Autodesk Inventor part; units mm, degrees
note: some values were not read from the file. Chosen so that the rebuilt part matches the saved one: bend side of "曲げパーツ2".
(part 2 of 2)
sketch "スケッチ2" plane through (0, 0, 0) normal (0, 0, -1) x (-1, 0, 0)
  line L0 (-121.1595, -137.1852) -> (-101.7935, -131.1964) projected
  arc A0 (-101.7935, -131.1964) -> (-101.8327, -129.2745) centre (-102.089, -130.2411) ccw projected
  line L1 (-101.8327, -129.2745) -> (-140.7437, -118.9579) projected
  arc A1 (-140.7437, -118.9579) -> (-142, -119.9245) centre (-141, -119.9245) ccw projected
  line L2 (-142, -119.9245) -> (-142, -142.2739) projected
  arc A2 (-142, -142.2739) -> (-140.7046, -143.2293) centre (-141, -142.2739) ccw projected
  line L3 (-140.7046, -143.2293) -> (-133.575, -141.0246) projected
  arc A3 (-133.575, -141.0246) -> (-132.8964, -140.2954) centre (-133.8705, -140.0692) ccw projected
  arc A4 (-126.6, -138) -> (-132.8964, -140.2954) centre (-129, -141.2) ccw projected
  arc A5 (-126.6, -138) -> (-126, -138.2) centre (-126, -137.2) ccw projected
  line L4 (-126, -138.2) -> (-125, -138.2) projected
  arc A6 (-125, -138.2) -> (-124.4, -138) centre (-125, -137.2) ccw projected
  arc A7 (-121.5639, -137.2238) -> (-124.4, -138) centre (-122, -141.2) ccw projected
  arc A8 (-121.5639, -137.2238) -> (-121.1595, -137.1852) centre (-121.4549, -136.2298) ccw projected
  line L5 (-125, 4) -> (-126, 4) projected
  arc A9 (-126, 4) -> (-126.6, 3.8) centre (-126, 3) ccw projected
  arc A10 (-132.8927, 6.0797) -> (-126.6, 3.8) centre (-129, 7) ccw projected
  arc A11 (-132.8927, 6.0797) -> (-133.5686, 6.8044) centre (-133.8659, 5.8496) ccw projected
  line L6 (-133.5686, 6.8044) -> (-140.7028, 9.0252) projected
  arc A12 (-140.7028, 9.0252) -> (-142, 8.0704) centre (-141, 8.0704) ccw projected
  line L7 (-142, 8.0704) -> (-142, -14.2755) projected
  arc A13 (-142, -14.2755) -> (-140.7437, -15.2421) centre (-141, -14.2755) ccw projected
  line L8 (-140.7437, -15.2421) -> (-101.9774, -4.9639) projected
  arc A14 (-101.9774, -4.9639) -> (-101.9364, -3.0425) centre (-102.2336, -3.9973) ccw projected
  line L9 (-101.9364, -3.0425) -> (-121.2641, 2.9741) projected
  arc A15 (-121.2641, 2.9741) -> (-121.6491, 3.0154) centre (-121.5614, 2.0193) ccw projected
  arc A16 (-124.4, 3.8) -> (-121.6491, 3.0154) centre (-122, 7) ccw projected
  arc A17 (-124.4, 3.8) -> (-125, 4) centre (-125, 3) ccw projected
  line L10 (-128.2505, -119.1666) -> (-93.3393, -128.4227) projected
  arc A18 (-93.3393, -128.4227) -> (-92.7876, -128.4114) centre (-93.0831, -127.4561) ccw projected
  line L11 (-92.7876, -128.4114) -> (-62.8561, -119.1554) projected
  arc A19 (-62.8561, -119.1554) -> (-63.1515, -117.2) centre (-63.1515, -118.2) ccw projected
  line L12 (-63.1515, -117.2) -> (-127.9942, -117.2) projected
  arc A20 (-127.9942, -117.2) -> (-128.2505, -119.1666) centre (-127.9942, -118.2) ccw projected
  line L13 (-127.9942, -17) -> (-63.676, -17) projected
  arc A21 (-63.676, -17) -> (-63.3788, -15.0452) centre (-63.676, -16) ccw projected
  line L14 (-63.3788, -15.0452) -> (-92.9626, -5.836) projected
  arc A22 (-92.9626, -5.836) -> (-93.5161, -5.8242) centre (-93.2598, -6.7908) ccw projected
  line L15 (-93.5161, -5.8242) -> (-128.2505, -15.0334) projected
  arc A23 (-128.2505, -15.0334) -> (-127.9942, -17) centre (-127.9942, -16) ccw projected
  line L16 (-52.2563, 5.1151) -> (-84.4313, -3.4155) projected
  arc A24 (-84.4313, -3.4155) -> (-84.4723, -5.337) centre (-84.1751, -4.3821) ccw projected
  line L17 (-84.4723, -5.337) -> (-52.2972, -15.3528) projected
  arc A25 (-52.2972, -15.3528) -> (-51, -14.398) centre (-52, -14.398) ccw projected
  line L18 (-51, -14.398) -> (-51, 4.1485) projected
  arc A26 (-51, 4.1485) -> (-52.2563, 5.1151) centre (-52, 4.1485) ccw projected
  line L19 (-51, -138.3485) -> (-51, -119.9851) projected
  arc A27 (-51, -119.9851) -> (-52.2954, -119.0297) centre (-52, -119.9851) ccw projected
  line L20 (-52.2954, -119.0297) -> (-84.2666, -128.9165) projected
  arc A28 (-84.2666, -128.9165) -> (-84.2275, -130.8385) centre (-83.9712, -129.8719) ccw projected
  line L21 (-84.2275, -130.8385) -> (-52.2563, -139.3151) projected
  arc A29 (-52.2563, -139.3151) -> (-51, -138.3485) centre (-52, -138.3485) ccw projected
  arc A30 (-86.4, 3.8) -> (-80.0808, 6.2) centre (-84, 7) ccw projected
  arc A31 (-86.4, 3.8) -> (-87, 4) centre (-87, 3) ccw projected
  line L22 (-87, 4) -> (-88, 4) projected
  arc A32 (-88, 4) -> (-88.6, 3.8) centre (-88, 3) ccw projected
  arc A33 (-95, 7) -> (-88.6, 3.8) centre (-91, 7) ccw projected
  line L23 (-95, 7) -> (-95, 10) projected
  arc A34 (-95, 10) -> (-96, 11) centre (-96, 10) ccw projected
  line L24 (-96, 11) -> (-117, 11) projected
  arc A35 (-117, 11) -> (-118, 10) centre (-117, 10) ccw projected
  line L25 (-118, 10) -> (-118, 7) projected
  arc A36 (-118.1024, 6.1007) -> (-118, 7) centre (-122, 7) ccw projected
  arc A37 (-118.1024, 6.1007) -> (-117.4252, 4.9211) centre (-117.128, 5.8759) ccw projected
  line L26 (-117.4252, 4.9211) -> (-93.4461, -2.5435) projected
  arc A38 (-93.4461, -2.5435) -> (-92.8926, -2.5553) centre (-93.1489, -1.5887) ccw projected
  line L27 (-92.8926, -2.5553) -> (-64.2705, 5.0334) projected
  arc A39 (-64.2705, 5.0334) -> (-64.5268, 7) centre (-64.5268, 6) ccw projected
  line L28 (-64.5268, 7) -> (-79.101, 7) projected
  arc A40 (-79.101, 7) -> (-80.0808, 6.2) centre (-79.101, 6) ccw projected
  line L29 (-117, -145.2) -> (-96, -145.2) projected
  arc A41 (-96, -145.2) -> (-95, -144.2) centre (-96, -144.2) ccw projected
  line L30 (-95, -144.2) -> (-95, -141.2) projected
  arc A42 (-88.6, -138) -> (-95, -141.2) centre (-91, -141.2) ccw projected
  arc A43 (-88.6, -138) -> (-88, -138.2) centre (-88, -137.2) ccw projected
  line L31 (-88, -138.2) -> (-87, -138.2) projected
  arc A44 (-87, -138.2) -> (-86.4, -138) centre (-87, -137.2) ccw projected
  arc A45 (-80.0808, -140.4) -> (-86.4, -138) centre (-84, -141.2) ccw projected
  arc A46 (-80.0808, -140.4) -> (-79.101, -141.2) centre (-79.101, -140.2) ccw projected
  line L32 (-79.101, -141.2) -> (-64.5268, -141.2) projected
  arc A47 (-64.5268, -141.2) -> (-64.2705, -139.2334) centre (-64.5268, -140.2) ccw projected
  line L33 (-64.2705, -139.2334) -> (-92.7208, -131.6903) projected
  arc A48 (-92.7208, -131.6903) -> (-93.2725, -131.7015) centre (-92.9771, -132.6569) ccw projected
  line L34 (-93.2725, -131.7015) -> (-117.413, -139.1668) projected
  arc A49 (-117.413, -139.1668) -> (-118.094, -140.3377) centre (-117.1176, -140.1221) ccw projected
  arc A50 (-118, -141.2) -> (-118.094, -140.3377) centre (-122, -141.2) ccw projected
  line L35 (-118, -141.2) -> (-118, -144.2) projected
  arc A51 (-118, -144.2) -> (-117, -145.2) centre (-117, -144.2) ccw projected
  line L36 (-123, -169.2) -> (-122, -169.2) projected
  arc A52 (-122, -169.2) -> (-121, -168.2) centre (-122, -168.2) ccw projected
  line L37 (-121, -168.2) -> (-121, -166.2) projected
  arc A53 (-121, -166.2) -> (-120.7896, -164.437) centre (-121.3519, -165.264) ccw projected
  line L38 (-120.7896, -164.437) -> (-128.9377, -158.8963) projected
  arc A54 (-128.9377, -158.8963) -> (-130.0623, -158.8963) centre (-129.5, -159.7232) ccw projected
  line L39 (-130.0623, -158.8963) -> (-135.1564, -162.3603) projected
  arc A55 (-135.1564, -162.3603) -> (-135.577, -163.3713) centre (-134.5941, -163.1872) ccw projected
  arc A56 (-135.575, -165.0182) -> (-135.577, -163.3713) centre (-140, -164.2) ccw projected
  arc A57 (-135.575, -165.0182) -> (-134.5917, -166.2) centre (-134.5917, -165.2) ccw projected
  line L40 (-134.5917, -166.2) -> (-134, -166.2) projected
  arc A58 (-134, -166.2) -> (-133.4, -166) centre (-134, -165.2) ccw projected
  arc A59 (-129.8, -165.3842) -> (-133.4, -166) centre (-131, -169.2) ccw projected
  arc A60 (-129.8, -165.3842) -> (-129.2, -165.3842) centre (-129.5, -164.4303) ccw projected
  arc A61 (-125.6, -166) -> (-129.2, -165.3842) centre (-128, -169.2) ccw projected
  arc A62 (-125.6, -166) -> (-125, -166.2) centre (-125, -165.2) ccw projected
  line L41 (-125, -166.2) -> (-124, -166.2) projected
  line L42 (-124, -166.2) -> (-124, -168.2) projected
  arc A63 (-124, -168.2) -> (-123, -169.2) centre (-123, -168.2) ccw projected
  line L43 (-121, 32) -> (-121, 34) projected
  arc A64 (-121, 34) -> (-122, 35) centre (-122, 34) ccw projected
  line L44 (-122, 35) -> (-123, 35) projected
  arc A65 (-123, 35) -> (-124, 34) centre (-123, 34) ccw projected
  line L45 (-124, 34) -> (-124, 32) projected
  line L46 (-124, 32) -> (-125, 32) projected
  arc A66 (-125, 32) -> (-125.6, 31.8) centre (-125, 31) ccw projected
  arc A67 (-129.2, 31.1842) -> (-125.6, 31.8) centre (-128, 35) ccw projected
  arc A68 (-129.2, 31.1842) -> (-129.8, 31.1842) centre (-129.5, 30.2303) ccw projected
  arc A69 (-133.4, 31.8) -> (-129.8, 31.1842) centre (-131, 35) ccw projected
  arc A70 (-133.4, 31.8) -> (-134, 32) centre (-134, 31) ccw projected
  line L47 (-134, 32) -> (-134.5917, 32) projected
  arc A71 (-134.5917, 32) -> (-135.575, 30.8182) centre (-134.5917, 31) ccw projected
  arc A72 (-135.577, 29.1713) -> (-135.575, 30.8182) centre (-140, 30) ccw projected
  arc A73 (-135.577, 29.1713) -> (-135.1564, 28.1603) centre (-134.5941, 28.9872) ccw projected
  line L48 (-135.1564, 28.1603) -> (-130.0623, 24.6963) projected
  arc A74 (-130.0623, 24.6963) -> (-128.9377, 24.6963) centre (-129.5, 25.5232) ccw projected
  line L49 (-128.9377, 24.6963) -> (-120.7896, 30.237) projected
  arc A75 (-120.7896, 30.237) -> (-121, 32) centre (-121.3519, 31.064) ccw projected
  line L50 (-125.6164, -157.5269) -> (-118.5623, -162.3237) projected
  arc A76 (-118.5623, -162.3237) -> (-117, -161.4968) centre (-118, -161.4968) ccw projected
  line L51 (-117, -161.4968) -> (-117, -151.9032) projected
  arc A77 (-117, -151.9032) -> (-118.5623, -151.0763) centre (-118, -151.9032) ccw projected
  line L52 (-118.5623, -151.0763) -> (-125.6164, -155.8731) projected
  arc A78 (-125.6164, -155.8731) -> (-125.6164, -157.5269) centre (-125.0541, -156.7) ccw projected
  line L53 (-117, 17.7032) -> (-117, 27.2968) projected
  arc A79 (-117, 27.2968) -> (-118.5623, 28.1237) centre (-118, 27.2968) ccw projected
  line L54 (-118.5623, 28.1237) -> (-125.6164, 23.3269) projected
  arc A80 (-125.6164, 23.3269) -> (-125.6164, 21.6731) centre (-125.0541, 22.5) ccw projected
  line L55 (-125.6164, 21.6731) -> (-118.5623, 16.8763) projected
  arc A81 (-118.5623, 16.8763) -> (-117, 17.7032) centre (-118, 17.7032) ccw projected
  line L56 (-122.9165, -148.2) -> (-136.0835, -148.2) projected
  arc A82 (-136.0835, -148.2) -> (-136.6458, -150.0269) centre (-136.0835, -149.2) ccw projected
  line L57 (-136.6458, -150.0269) -> (-130.0623, -154.5037) projected
  arc A83 (-130.0623, -154.5037) -> (-128.9377, -154.5037) centre (-129.5, -153.6768) ccw projected
  line L58 (-128.9377, -154.5037) -> (-122.3542, -150.0269) projected
  arc A84 (-122.3542, -150.0269) -> (-122.9165, -148.2) centre (-122.9165, -149.2) ccw projected
  line L59 (-130.0623, 20.3037) -> (-136.6458, 15.8269) projected
  arc A85 (-136.6458, 15.8269) -> (-136.0835, 14) centre (-136.0835, 15) ccw projected
  line L60 (-136.0835, 14) -> (-122.9165, 14) projected
  arc A86 (-122.9165, 14) -> (-122.3542, 15.8269) centre (-122.9165, 15) ccw projected
  line L61 (-122.3542, 15.8269) -> (-128.9377, 20.3037) projected
  arc A87 (-128.9377, 20.3037) -> (-130.0623, 20.3037) centre (-129.5, 19.4768) ccw projected
  line L62 (-140.4377, 16.8763) -> (-133.3836, 21.6731) projected
  arc A88 (-133.3836, 21.6731) -> (-133.3836, 23.3269) centre (-133.9459, 22.5) ccw projected
  line L63 (-133.3836, 23.3269) -> (-137.0951, 25.8507) projected
  arc A89 (-137.0951, 25.8507) -> (-138.0834, 25.9286) centre (-137.6574, 25.0238) ccw projected
  arc A90 (-140.8182, 25.575) -> (-138.0834, 25.9286) centre (-140, 30) ccw projected
  arc A91 (-140.8182, 25.575) -> (-142, 24.5917) centre (-141, 24.5917) ccw projected
  line L64 (-142, 24.5917) -> (-142, 17.7032) projected
  arc A92 (-142, 17.7032) -> (-140.4377, 16.8763) centre (-141, 17.7032) ccw projected
  arc A93 (-138.0834, -160.1286) -> (-140.8182, -159.775) centre (-140, -164.2) ccw projected
  arc A94 (-138.0834, -160.1286) -> (-137.0951, -160.0507) centre (-137.6574, -159.2238) ccw projected
  line L65 (-137.0951, -160.0507) -> (-133.3836, -157.5269) projected
  arc A95 (-133.3836, -157.5269) -> (-133.3836, -155.8731) centre (-133.9459, -156.7) ccw projected
  line L66 (-133.3836, -155.8731) -> (-140.4377, -151.0763) projected
  arc A96 (-140.4377, -151.0763) -> (-142, -151.9032) centre (-141, -151.9032) ccw projected
  line L67 (-142, -151.9032) -> (-142, -158.7917) projected
  arc A97 (-142, -158.7917) -> (-140.8182, -159.775) centre (-141, -158.7917) ccw projected
  line L68 (-83, -144.2) -> (-83, -141.2) projected
  arc A98 (-83, -141.2) -> (-85, -141.2) centre (-84, -141.2) ccw projected
  line L69 (-85, -141.2) -> (-90, -141.2) projected
  arc A99 (-90, -141.2) -> (-92, -141.2) centre (-91, -141.2) ccw projected
  line L70 (-92, -141.2) -> (-92, -144.2) projected
  arc A100 (-92, -144.2) -> (-90, -144.2) centre (-91, -144.2) ccw projected
  line L71 (-90, -144.2) -> (-85, -144.2) projected
  arc A101 (-85, -144.2) -> (-83, -144.2) centre (-84, -144.2) ccw projected
  line L72 (-121, 7) -> (-121, 10) projected
  arc A102 (-121, 10) -> (-123, 10) centre (-122, 10) ccw projected
  line L73 (-123, 10) -> (-128, 10) projected
  arc A103 (-128, 10) -> (-130, 10) centre (-129, 10) ccw projected
  line L74 (-130, 10) -> (-130, 7) projected
  arc A104 (-130, 7) -> (-128, 7) centre (-129, 7) ccw projected
  line L75 (-128, 7) -> (-123, 7) projected
  arc A105 (-123, 7) -> (-121, 7) centre (-122, 7) ccw projected
  line L76 (-90, 7) -> (-85, 7) projected
  arc A106 (-85, 7) -> (-83, 7) centre (-84, 7) ccw projected
  line L77 (-83, 7) -> (-83, 10) projected
  arc A107 (-83, 10) -> (-85, 10) centre (-84, 10) ccw projected
  line L78 (-85, 10) -> (-90, 10) projected
  arc A108 (-90, 10) -> (-92, 10) centre (-91, 10) ccw projected
  line L79 (-92, 10) -> (-92, 7) projected
  arc A109 (-92, 7) -> (-90, 7) centre (-91, 7) ccw projected
  line L80 (-128, -144.2) -> (-123, -144.2) projected
  arc A110 (-123, -144.2) -> (-121, -144.2) centre (-122, -144.2) ccw projected
  line L81 (-121, -144.2) -> (-121, -141.2) projected
  arc A111 (-121, -141.2) -> (-123, -141.2) centre (-122, -141.2) ccw projected
  line L82 (-123, -141.2) -> (-128, -141.2) projected
  arc A112 (-128, -141.2) -> (-130, -141.2) centre (-129, -141.2) ccw projected
  line L83 (-130, -141.2) -> (-130, -144.2) projected
  arc A113 (-130, -144.2) -> (-128, -144.2) centre (-129, -144.2) ccw projected
  circle A114 centre (-140, -164.2) radius 1.5 projected
  circle A115 centre (-140, 30) radius 1.5 projected
  arc A116 (-136.7273, 33.0886) -> (-136.9114, 33.2727) centre (-140, 30) ccw projected
  arc A117 (-136.7273, 33.0886) -> (-135, 33.7749) centre (-136, 33.7749) ccw projected
  line L84 (-135, 33.7749) -> (-135, 34) projected
  arc A118 (-135, 34) -> (-136, 35) centre (-136, 34) ccw projected
  line L85 (-136, 35) -> (-136.2251, 35) projected
  arc A119 (-136.2251, 35) -> (-136.9114, 33.2727) centre (-136.2251, 34) ccw projected
  line L86 (-136.2251, -169.2) -> (-136, -169.2) projected
  arc A120 (-136, -169.2) -> (-135, -168.2) centre (-136, -168.2) ccw projected
  line L87 (-135, -168.2) -> (-135, -167.9749) projected
  arc A121 (-135, -167.9749) -> (-136.7273, -167.2886) centre (-136, -167.9749) ccw projected
  arc A122 (-136.9114, -167.4727) -> (-136.7273, -167.2886) centre (-140, -164.2) ccw projected
  arc A123 (-136.9114, -167.4727) -> (-136.2251, -169.2) centre (-136.2251, -168.2) ccw projected
  line L88 (-79, 10) -> (-48, 10) projected
  line L89 (-48, 10) -> (-48, -144.2) projected
  line L90 (-48, -144.2) -> (-79, -144.2) projected
  arc A124 (-79, -144.2) -> (-80, -145.2) centre (-79, -145.2) ccw projected
  line L91 (-80, -145.2) -> (-80, -148.2) projected
  line L92 (-80, -148.2) -> (-113, -148.2) projected
  arc A125 (-113, -148.2) -> (-114, -149.2) centre (-113, -149.2) ccw projected
  line L93 (-114, -149.2) -> (-114, -169.2) projected
  line L94 (-114, -169.2) -> (-116, -169.2) projected
  arc A126 (-116, -169.2) -> (-118, -169.2) centre (-117, -169.2) ccw projected
  line L95 (-118, -169.2) -> (-118, -172.2) projected
  line L96 (-118, -172.2) -> (-127, -172.2) projected
  line L97 (-127, -172.2) -> (-127, -169.2) projected
  arc A127 (-127, -169.2) -> (-129, -169.2) centre (-128, -169.2) ccw projected
  line L98 (-129, -169.2) -> (-130, -169.2) projected
  arc A128 (-130, -169.2) -> (-132, -169.2) centre (-131, -169.2) ccw projected
  line L99 (-132, -169.2) -> (-132, -172.2) projected
  line L100 (-132, -172.2) -> (-141, -172.2) projected
  line L101 (-141, -172.2) -> (-141, -169.2) projected
  arc A129 (-141, -169.2) -> (-143, -169.2) centre (-142, -169.2) ccw projected
  line L102 (-143, -169.2) -> (-145, -169.2) projected
  line L103 (-145, -169.2) -> (-145, 35) projected
  line L104 (-145, 35) -> (-143, 35) projected
  arc A130 (-143, 35) -> (-141, 35) centre (-142, 35) ccw projected
  line L105 (-141, 35) -> (-141, 38) projected
  line L106 (-141, 38) -> (-132, 38) projected
  line L107 (-132, 38) -> (-132, 35) projected
  arc A131 (-132, 35) -> (-130, 35) centre (-131, 35) ccw projected
  line L108 (-130, 35) -> (-129, 35) projected
  arc A132 (-129, 35) -> (-127, 35) centre (-128, 35) ccw projected
  line L109 (-127, 35) -> (-127, 38) projected
  line L110 (-127, 38) -> (-118, 38) projected
  line L111 (-118, 38) -> (-118, 35) projected
  arc A133 (-118, 35) -> (-116, 35) centre (-117, 35) ccw projected
  line L112 (-116, 35) -> (-114, 35) projected
  line L113 (-114, 35) -> (-114, 15) projected
  arc A134 (-114, 15) -> (-113, 14) centre (-113, 15) ccw projected
  line L114 (-113, 14) -> (-80, 14) projected
  line L115 (-80, 14) -> (-80, 11) projected
  arc A135 (-80, 11) -> (-79, 10) centre (-79, 11) ccw projected
  point P0 (0, 0)
extrude "押し出し2" add sketch "スケッチ2" against normal blind 0.5 contours A8 A7 A6 L4 A5 A4 A3 L3 A2 L2 A1 L1 A0 L0 | A17 A16 A15 L9 A14 L8 A13 L7 A12 L6 A11 A10 A9 L5 | A20 L12 A19 L11 A18 L10 | A23 L15 A22 L14 A21 L13 | A26 L18 A25 L17 A24 L16 | A29 L21 A28 L20 A27 L19 | A30 A40 L28 A39 L27 A38 L26 A37 A36 L25 A35 L24 A34 L23 A33 A32 L22 A31 | A51 L35 A50 A49 L34 A48 L33 A47 L32 A46 A45 A44 L31 A43 A42 L30 A41 L29 | A63 L42 L41 A62 A61 A60 A59 A58 L40 A57 A56 A55 L39 A54 L38 A53 L37 A52 L36 | A75 L49 A74 L48 A73 A72 A71 L47 A70 A69 A68 A67 A66 L46 L45 A65 L44 A64 L43 | A78 L52 A77 L51 A76 L50 | A81 L55 A80 L54 A79 L53 | A84 L58 A83 L57 A82 L56 | A87 L61 A86 L60 A85 L59 | A92 L64 A91 A90 A89 L63 A88 L62 | A93 A97 L67 A96 L66 A95 L65 A94 | A116 A119 L85 A118 L84 A117 | A123 A122 A121 L87 A120 L86
sketch "スケッチ3" plane through (0, 0, 2) normal (0, 0, 1) x (1, 0, 0)
  circle A0 centre (-34.5, -35.6) radius 1.5
  line L0 (-34.5, -34.1) -> (-29, -34.1)
  arc A1 (-29, -34.1) -> (-27, -34.1) centre (-28, -34.1) ccw
  line L1 (-27, -34.1) -> (-27, -31.1)
  arc A2 (-27, -31.1) -> (-29, -31.1) centre (-28, -31.1) ccw
  line L2 (-29, -31.1) -> (-40, -31.1)
  arc A3 (-40, -31.1) -> (-42, -31.1) centre (-41, -31.1) ccw
  line L3 (-42, -31.1) -> (-42, -34.1)
  arc A4 (-42, -34.1) -> (-40, -34.1) centre (-41, -34.1) ccw
  line L4 (-40, -34.1) -> (-34.5, -34.1)
  line L5 (40, -52.1) -> (29, -52.1)
  arc A5 (29, -52.1) -> (27, -52.1) centre (28, -52.1) ccw
  line L6 (27, -52.1) -> (27, -55.1)
  arc A6 (27, -55.1) -> (29, -55.1) centre (28, -55.1) ccw
  line L7 (29, -55.1) -> (34.5, -55.1)
  circle A7 centre (34.5, -56.6) radius 1.5
  line L8 (34.5, -55.1) -> (40, -55.1)
  arc A8 (40, -55.1) -> (42, -55.1) centre (41, -55.1) ccw
  line L9 (42, -55.1) -> (42, -52.1)
  arc A9 (42, -52.1) -> (40, -52.1) centre (41, -52.1) ccw
  arc A10 (-36.9671, -20) -> (-34.9671, -20) centre (-35.9671, -20) ccw
  line L10 (-34.9671, -20) -> (-29.4671, -20)
  circle A11 centre (-29.4671, -21.5) radius 1.5
  line L11 (-29.4671, -20) -> (-23.9671, -20)
  arc A12 (-23.9671, -20) -> (-21.9671, -20) centre (-22.9671, -20) ccw
  line L12 (-21.9671, -20) -> (-21.9671, -17)
  arc A13 (-21.9671, -17) -> (-23.9671, -17) centre (-22.9671, -17) ccw
  line L13 (-23.9671, -17) -> (-34.9671, -17)
  arc A14 (-34.9671, -17) -> (-36.9671, -17) centre (-35.9671, -17) ccw
  line L14 (-36.9671, -17) -> (-36.9671, -20)
  line L15 (5.4918, -114.1907) -> (-0.0082, -114.1907)
  circle A15 centre (-0.0082, -112.6907) radius 1.5
  line L16 (-0.0082, -114.1907) -> (-5.5082, -114.1907)
  arc A16 (-5.5082, -114.1907) -> (-7.5082, -114.1907) centre (-6.5082, -114.1907) ccw
  line L17 (-7.5082, -114.1907) -> (-7.5082, -117.1907)
  arc A17 (-7.5082, -117.1907) -> (-5.5082, -117.1907) centre (-6.5082, -117.1907) ccw
  line L18 (-5.5082, -117.1907) -> (5.4918, -117.1907)
  arc A18 (5.4918, -117.1907) -> (7.4918, -117.1907) centre (6.4918, -117.1907) ccw
  line L19 (7.4918, -117.1907) -> (7.4918, -114.1907)
  arc A19 (7.4918, -114.1907) -> (5.4918, -114.1907) centre (6.4918, -114.1907) ccw
  line L20 (7.5, -20) -> (7.5, -17)
  arc A20 (7.5, -17) -> (5.5, -17) centre (6.5, -17) ccw
  line L21 (5.5, -17) -> (-5.5, -17)
  arc A21 (-5.5, -17) -> (-7.5, -17) centre (-6.5, -17) ccw
  line L22 (-7.5, -17) -> (-7.5, -20)
  arc A22 (-7.5, -20) -> (-5.5, -20) centre (-6.5, -20) ccw
  line L23 (-5.5, -20) -> (0, -20)
  circle A23 centre (0, -21.5) radius 1.5
  line L24 (0, -20) -> (5.5, -20)
  arc A24 (5.5, -20) -> (7.5, -20) centre (6.5, -20) ccw
  arc A25 (-34.9671, -114.2) -> (-36.9671, -114.2) centre (-35.9671, -114.2) ccw
  line L25 (-36.9671, -114.2) -> (-36.9671, -117.2)
  arc A26 (-36.9671, -117.2) -> (-34.9671, -117.2) centre (-35.9671, -117.2) ccw
  line L26 (-34.9671, -117.2) -> (-23.9671, -117.2)
  arc A27 (-23.9671, -117.2) -> (-21.9671, -117.2) centre (-22.9671, -117.2) ccw
  line L27 (-21.9671, -117.2) -> (-21.9671, -114.2)
  arc A28 (-21.9671, -114.2) -> (-23.9671, -114.2) centre (-22.9671, -114.2) ccw
  line L28 (-23.9671, -114.2) -> (-29.4671, -114.2)
  circle A29 centre (-29.4671, -112.7) radius 1.5
  line L29 (-29.4671, -114.2) -> (-34.9671, -114.2)
  line L30 (47.8619, -113.9653) -> (45.29, -109.593)
  arc A30 (45.29, -109.593) -> (44.4281, -109.1) centre (44.4281, -110.1) ccw
  line L31 (44.4281, -109.1) -> (15.2527, -109.1)
  arc A31 (15.2527, -109.1) -> (14.3908, -109.593) centre (15.2527, -110.1) ccw
  line L32 (14.3908, -109.593) -> (11.8189, -113.9653)
  arc A32 (11.8189, -113.9653) -> (11.6808, -114.4723) centre (12.6808, -114.4723) ccw
  line L33 (11.6808, -114.4723) -> (11.6808, -117.2)
  line L34 (11.6808, -117.2) -> (11.399, -117.2)
  arc A33 (11.399, -117.2) -> (10.4192, -118) centre (11.399, -118.2) ccw
  arc A34 (4.1, -120.4) -> (10.4192, -118) centre (6.5, -117.2) ccw
  arc A35 (4.1, -120.4) -> (3.5, -120.2) centre (3.5, -121.2) ccw
  line L35 (3.5, -120.2) -> (-3.5, -120.2)
  arc A36 (-3.5, -120.2) -> (-4.1, -120.4) centre (-3.5, -121.2) ccw
  arc A37 (-10.4192, -118) -> (-4.1, -120.4) centre (-6.5, -117.2) ccw
  arc A38 (-10.4192, -118) -> (-11.399, -117.2) centre (-11.399, -118.2) ccw
  line L36 (-11.399, -117.2) -> (-11.6808, -117.2)
  line L37 (-11.6808, -117.2) -> (-11.6808, -115.2)
  arc A39 (-11.6808, -115.2) -> (-12.6808, -114.2) centre (-12.6808, -115.2) ccw
  line L38 (-12.6808, -114.2) -> (-16.7863, -114.2)
  arc A40 (-16.7863, -114.2) -> (-17.7863, -115.2) centre (-16.7863, -115.2) ccw
  line L39 (-17.7863, -115.2) -> (-17.7863, -117.2)
  line L40 (-17.7863, -117.2) -> (-18.0681, -117.2)
  arc A41 (-18.0681, -117.2) -> (-19.0479, -118) centre (-18.0681, -118.2) ccw
  arc A42 (-25.3671, -120.4) -> (-19.0479, -118) centre (-22.9671, -117.2) ccw
  arc A43 (-25.3671, -120.4) -> (-25.9671, -120.2) centre (-25.9671, -121.2) ccw
  line L41 (-25.9671, -120.2) -> (-32.9671, -120.2)
  arc A44 (-32.9671, -120.2) -> (-33.5671, -120.4) centre (-32.9671, -121.2) ccw
  arc A45 (-39.8862, -118) -> (-33.5671, -120.4) centre (-35.9671, -117.2) ccw
  arc A46 (-39.8862, -118) -> (-40.866, -117.2) centre (-40.866, -118.2) ccw
  line L42 (-40.866, -117.2) -> (-41.1478, -117.2)
  line L43 (-41.1478, -117.2) -> (-41.1478, -115.2)
  arc A47 (-41.1478, -115.2) -> (-42.1478, -114.2) centre (-42.1478, -115.2) ccw
  line L44 (-42.1478, -114.2) -> (-52, -114.2)
  line L45 (-52, -114.2) -> (-52, -20)
  line L46 (-52, -20) -> (-42.1478, -20)
  arc A48 (-42.1478, -20) -> (-41.1478, -19) centre (-42.1478, -19) ccw
  line L47 (-41.1478, -19) -> (-41.1478, -17)
  line L48 (-41.1478, -17) -> (-40.866, -17)
  arc A49 (-40.866, -17) -> (-39.8862, -16.2) centre (-40.866, -16) ccw
  arc A50 (-33.5671, -13.8) -> (-39.8862, -16.2) centre (-35.9671, -17) ccw
  arc A51 (-33.5671, -13.8) -> (-32.9671, -14) centre (-32.9671, -13) ccw
  line L49 (-32.9671, -14) -> (-25.9671, -14)
  arc A52 (-25.9671, -14) -> (-25.3671, -13.8) centre (-25.9671, -13) ccw
  arc A53 (-19.0479, -16.2) -> (-25.3671, -13.8) centre (-22.9671, -17) ccw
  arc A54 (-19.0479, -16.2) -> (-18.0681, -17) centre (-18.0681, -16) ccw
  line L50 (-18.0681, -17) -> (-17.7863, -17)
  line L51 (-17.7863, -17) -> (-17.7863, -19)
  arc A55 (-17.7863, -19) -> (-16.7863, -20) centre (-16.7863, -19) ccw
  line L52 (-16.7863, -20) -> (-12.6808, -20)
  arc A56 (-12.6808, -20) -> (-11.6808, -19) centre (-12.6808, -19) ccw
  line L53 (-11.6808, -19) -> (-11.6808, -17)
  line L54 (-11.6808, -17) -> (-11.399, -17)
  arc A57 (-11.399, -17) -> (-10.4192, -16.2) centre (-11.399, -16) ccw
  arc A58 (-4.1, -13.8) -> (-10.4192, -16.2) centre (-6.5, -17) ccw
  arc A59 (-4.1, -13.8) -> (-3.5, -14) centre (-3.5, -13) ccw
  line L55 (-3.5, -14) -> (3.5, -14)
  arc A60 (3.5, -14) -> (4.1, -13.8) centre (3.5, -13) ccw
  arc A61 (10.4192, -16.2) -> (4.1, -13.8) centre (6.5, -17) ccw
  arc A62 (10.4192, -16.2) -> (11.399, -17) centre (11.399, -16) ccw
  line L56 (11.399, -17) -> (11.6808, -17)
  line L57 (11.6808, -17) -> (11.6808, -19.7277)
  arc A63 (11.6808, -19.7277) -> (11.8189, -20.2347) centre (12.6808, -19.7277) ccw
  line L58 (11.8189, -20.2347) -> (14.3908, -24.607)
  arc A64 (14.3908, -24.607) -> (15.2527, -25.1) centre (15.2527, -24.1) ccw
  line L59 (15.2527, -25.1) -> (44.4281, -25.1)
  arc A65 (44.4281, -25.1) -> (45.29, -24.607) centre (44.4281, -24.1) ccw
  line L60 (45.29, -24.607) -> (47.8619, -20.2347)
  arc A66 (47.8619, -20.2347) -> (48, -19.7277) centre (47, -19.7277) ccw
  line L61 (48, -19.7277) -> (48, 14)
  line L62 (48, 14) -> (145, 14)
  line L63 (145, 14) -> (145, -148.2)
  line L64 (145, -148.2) -> (48, -148.2)
  line L65 (48, -148.2) -> (48, -114.4723)
  arc A67 (48, -114.4723) -> (47.8619, -113.9653) centre (47, -114.4723) ccw
  arc A68 (27.001, -34.1451) -> (29, -34.1) centre (28, -34.1) ccw
  line L66 (29, -34.1) -> (40, -34.1)
  arc A69 (40, -34.1) -> (42, -34.1) centre (41, -34.1) ccw
  line L67 (42, -34.1) -> (42, -31.1)
  arc A70 (42, -31.1) -> (40, -31.1) centre (41, -31.1) ccw
  line L68 (40, -31.1) -> (34.5, -31.1)
  circle A71 centre (34.5, -29.6) radius 1.5
  line L69 (34.5, -31.1) -> (29, -31.1)
  arc A72 (29, -31.1) -> (27, -31.1) centre (28, -31.1) ccw
  line L70 (27, -31.1) -> (27, -32.5348)
  line L71 (27.5466, -33.9316) -> (27, -32.5348)
  line L72 (27.001, -34.1451) -> (27.5466, -33.9316)
  line L73 (-29, -52.1) -> (-40, -52.1)
  arc A73 (-40, -52.1) -> (-42, -52.1) centre (-41, -52.1) ccw
  line L74 (-42, -52.1) -> (-42, -55.1)
  arc A74 (-42, -55.1) -> (-40, -55.1) centre (-41, -55.1) ccw
  line L75 (-40, -55.1) -> (-34.5, -55.1)
  circle A75 centre (-34.5, -56.6) radius 1.5
  line L76 (-34.5, -55.1) -> (-29, -55.1)
  arc A76 (-29, -55.1) -> (-27, -55.1) centre (-28, -55.1) ccw
  line L77 (-27, -55.1) -> (-27, -52.1)
  arc A77 (-27, -52.1) -> (-29, -52.1) centre (-28, -52.1) ccw
  arc A78 (90, -144.2) -> (92, -144.2) centre (91, -144.2) ccw
  line L78 (92, -144.2) -> (92, -141.2)
  arc A79 (92, -141.2) -> (90, -141.2) centre (91, -141.2) ccw
  line L79 (90, -141.2) -> (85, -141.2)
  arc A80 (85, -141.2) -> (83, -141.2) centre (84, -141.2) ccw
  line L80 (83, -141.2) -> (83, -144.2)
  arc A81 (83, -144.2) -> (85, -144.2) centre (84, -144.2) ccw
  line L81 (85, -144.2) -> (90, -144.2)
  arc A82 (123, 10) -> (121, 10) centre (122, 10) ccw
  line L82 (121, 10) -> (121, 7)
  arc A83 (121, 7) -> (123, 7) centre (122, 7) ccw
  line L83 (123, 7) -> (128, 7)
  arc A84 (128, 7) -> (130, 7) centre (129, 7) ccw
  line L84 (130, 7) -> (130, 10)
  arc A85 (130, 10) -> (128, 10) centre (129, 10) ccw
  line L85 (128, 10) -> (123, 10)
  arc A86 (85, 10) -> (83, 10) centre (84, 10) ccw
  line L86 (83, 10) -> (83, 7)
  arc A87 (83, 7) -> (85, 7) centre (84, 7) ccw
  line L87 (85, 7) -> (90, 7)
  arc A88 (90, 7) -> (92, 7) centre (91, 7) ccw
  line L88 (92, 7) -> (92, 10)
  arc A89 (92, 10) -> (90, 10) centre (91, 10) ccw
  line L89 (90, 10) -> (85, 10)
  arc A90 (123, -141.2) -> (121, -141.2) centre (122, -141.2) ccw
  line L90 (121, -141.2) -> (121, -144.2)
  arc A91 (121, -144.2) -> (123, -144.2) centre (122, -144.2) ccw
  line L91 (123, -144.2) -> (128, -144.2)
  arc A92 (128, -144.2) -> (130, -144.2) centre (129, -144.2) ccw
  line L92 (130, -144.2) -> (130, -141.2)
  arc A93 (130, -141.2) -> (128, -141.2) centre (129, -141.2) ccw
  line L93 (128, -141.2) -> (123, -141.2)
  line L94 (48, -20) -> (145, -20)
  line L95 (48, -114.2) -> (145, -114.2)
  line L96 (145, 14) -> (48, 14)
  line L97 (80, 14) -> (80, 10)
  line L98 (48, 14) -> (48, -19.7277)
  line L99 (48, 10) -> (80, 10)
  line L100 (80, -114.2) -> (80, -144.2)
  line L101 (48, -144.2) -> (80, -144.2)
  line L102 (80, 10) -> (80, -20)
  line L103 (80, -144.2) -> (80, -148.2)
  line L104 (80, 10) -> (100, 14)
  line L105 (48, 14) -> (145, 14)
  line L106 (80, -144.2) -> (100, -148.2)
  line L107 (48, -148.2) -> (145, -148.2)
  point P0 (0, 0)
  point P1 (0, 0)
  dimension "d4" = 3
  dimension "d5" = 3
  dimension "d6" = 20
  dimension "d7" = 20
  constraints: 216 end point, 172 point on circle, 86 centre point, 10 point on line, 8 vertical alignment, 6 perpendicular, 2 vertical, 8 other
  measures "d4" distance between parallel lines of L86 L97
  measures "d5" distance between parallel lines of L100 L80
  measures "d6" distance from line of L97 L104.end
  measures "d7" distance from line of L106.end L103
sketch "スケッチ4" plane through (0, 0, 2) normal (0, 0, 1) x (1, 0, 0)
  arc A0 (140.7437, -15.2421) -> (142, -14.2755) centre (141, -14.2755) ccw projected
  line L0 (142, -14.2755) -> (142, 8.0704) projected
  arc A1 (142, 8.0704) -> (140.7028, 9.0252) centre (141, 8.0704) ccw projected
  line L1 (140.7028, 9.0252) -> (133.5686, 6.8044) projected
  arc A2 (133.5686, 6.8044) -> (132.8927, 6.0797) centre (133.8659, 5.8496) ccw projected
  arc A3 (126.6, 3.8) -> (132.8927, 6.0797) centre (129, 7) ccw projected
  arc A4 (126.6, 3.8) -> (126, 4) centre (126, 3) ccw projected
  line L2 (126, 4) -> (125, 4) projected
  arc A5 (125, 4) -> (124.4, 3.8) centre (125, 3) ccw projected
  arc A6 (121.6491, 3.0154) -> (124.4, 3.8) centre (122, 7) ccw projected
  arc A7 (121.6491, 3.0154) -> (121.2641, 2.9741) centre (121.5614, 2.0193) ccw projected
  line L3 (121.2641, 2.9741) -> (101.9364, -3.0425) projected
  arc A8 (101.9364, -3.0425) -> (101.9774, -4.9639) centre (102.2336, -3.9973) ccw projected
  line L4 (101.9774, -4.9639) -> (140.7437, -15.2421) projected
  arc A9 (93.5161, -5.8242) -> (92.9626, -5.836) centre (93.2598, -6.7908) ccw projected
  line L5 (92.9626, -5.836) -> (63.3788, -15.0452) projected
  arc A10 (63.3788, -15.0452) -> (63.676, -17) centre (63.676, -16) ccw projected
  line L6 (63.676, -17) -> (127.9942, -17) projected
  arc A11 (127.9942, -17) -> (128.2505, -15.0334) centre (127.9942, -16) ccw projected
  line L7 (128.2505, -15.0334) -> (93.5161, -5.8242) projected
  arc A12 (84.2275, -130.8385) -> (84.2666, -128.9165) centre (83.9712, -129.8719) ccw projected
  line L8 (84.2666, -128.9165) -> (52.2954, -119.0297) projected
  arc A13 (52.2954, -119.0297) -> (51, -119.9851) centre (52, -119.9851) ccw projected
  line L9 (51, -119.9851) -> (51, -138.3485) projected
  arc A14 (51, -138.3485) -> (52.2563, -139.3151) centre (52, -138.3485) ccw projected
  line L10 (52.2563, -139.3151) -> (84.2275, -130.8385) projected
  line L11 (64.5268, -141.2) -> (79.101, -141.2) projected
  arc A15 (79.101, -141.2) -> (80.0808, -140.4) centre (79.101, -140.2) ccw projected
  arc A16 (86.4, -138) -> (80.0808, -140.4) centre (84, -141.2) ccw projected
  arc A17 (86.4, -138) -> (87, -138.2) centre (87, -137.2) ccw projected
  line L12 (87, -138.2) -> (88, -138.2) projected
  arc A18 (88, -138.2) -> (88.6, -138) centre (88, -137.2) ccw projected
  arc A19 (95, -141.2) -> (88.6, -138) centre (91, -141.2) ccw projected
  line L13 (95, -141.2) -> (95, -144.2) projected
  arc A20 (95, -144.2) -> (96, -145.2) centre (96, -144.2) ccw projected
  line L14 (96, -145.2) -> (117, -145.2) projected
  arc A21 (117, -145.2) -> (118, -144.2) centre (117, -144.2) ccw projected
  line L15 (118, -144.2) -> (118, -141.2) projected
  arc A22 (118.094, -140.3377) -> (118, -141.2) centre (122, -141.2) ccw projected
  arc A23 (118.094, -140.3377) -> (117.413, -139.1668) centre (117.1176, -140.1221) ccw projected
  line L16 (117.413, -139.1668) -> (93.2725, -131.7015) projected
  arc A24 (93.2725, -131.7015) -> (92.7208, -131.6903) centre (92.9771, -132.6569) ccw projected
  line L17 (92.7208, -131.6903) -> (64.2705, -139.2334) projected
  arc A25 (64.2705, -139.2334) -> (64.5268, -141.2) centre (64.5268, -140.2) ccw projected
  arc A26 (134.5917, -166.2) -> (135.575, -165.0182) centre (134.5917, -165.2) ccw projected
  arc A27 (135.577, -163.3713) -> (135.575, -165.0182) centre (140, -164.2) ccw projected
  arc A28 (135.577, -163.3713) -> (135.1564, -162.3603) centre (134.5941, -163.1872) ccw projected
  line L18 (135.1564, -162.3603) -> (130.0623, -158.8963) projected
  arc A29 (130.0623, -158.8963) -> (128.9377, -158.8963) centre (129.5, -159.7232) ccw projected
  line L19 (128.9377, -158.8963) -> (120.7896, -164.437) projected
  arc A30 (120.7896, -164.437) -> (121, -166.2) centre (121.3519, -165.264) ccw projected
  line L20 (121, -166.2) -> (121, -168.2) projected
  arc A31 (121, -168.2) -> (122, -169.2) centre (122, -168.2) ccw projected
  line L21 (122, -169.2) -> (123, -169.2) projected
  arc A32 (123, -169.2) -> (124, -168.2) centre (123, -168.2) ccw projected
  line L22 (124, -168.2) -> (124, -166.2) projected
  line L23 (124, -166.2) -> (125, -166.2) projected
  arc A33 (125, -166.2) -> (125.6, -166) centre (125, -165.2) ccw projected
  arc A34 (129.2, -165.3842) -> (125.6, -166) centre (128, -169.2) ccw projected
  arc A35 (129.2, -165.3842) -> (129.8, -165.3842) centre (129.5, -164.4303) ccw projected
  arc A36 (133.4, -166) -> (129.8, -165.3842) centre (131, -169.2) ccw projected
  arc A37 (133.4, -166) -> (134, -166.2) centre (134, -165.2) ccw projected
  line L24 (134, -166.2) -> (134.5917, -166.2) projected
  arc A38 (118.5623, -151.0763) -> (117, -151.9032) centre (118, -151.9032) ccw projected
  line L25 (117, -151.9032) -> (117, -161.4968) projected
  arc A39 (117, -161.4968) -> (118.5623, -162.3237) centre (118, -161.4968) ccw projected
  line L26 (118.5623, -162.3237) -> (125.6164, -157.5269) projected
  arc A40 (125.6164, -157.5269) -> (125.6164, -155.8731) centre (125.0541, -156.7) ccw projected
  line L27 (125.6164, -155.8731) -> (118.5623, -151.0763) projected
  arc A41 (128.9377, -154.5037) -> (130.0623, -154.5037) centre (129.5, -153.6768) ccw projected
  line L28 (130.0623, -154.5037) -> (136.6458, -150.0269) projected
  arc A42 (136.6458, -150.0269) -> (136.0835, -148.2) centre (136.0835, -149.2) ccw projected
  line L29 (136.0835, -148.2) -> (122.9165, -148.2) projected
  arc A43 (122.9165, -148.2) -> (122.3542, -150.0269) centre (122.9165, -149.2) ccw projected
  line L30 (122.3542, -150.0269) -> (128.9377, -154.5037) projected
  arc A44 (138.0834, 25.9286) -> (140.8182, 25.575) centre (140, 30) ccw projected
  arc A45 (138.0834, 25.9286) -> (137.0951, 25.8507) centre (137.6574, 25.0238) ccw projected
  line L31 (137.0951, 25.8507) -> (133.3836, 23.3269) projected
  arc A46 (133.3836, 23.3269) -> (133.3836, 21.6731) centre (133.9459, 22.5) ccw projected
  line L32 (133.3836, 21.6731) -> (140.4377, 16.8763) projected
  arc A47 (140.4377, 16.8763) -> (142, 17.7032) centre (141, 17.7032) ccw projected
  line L33 (142, 17.7032) -> (142, 24.5917) projected
  arc A48 (142, 24.5917) -> (140.8182, 25.575) centre (141, 24.5917) ccw projected
  arc A49 (136, 35) -> (135, 34) centre (136, 34) ccw projected
  line L34 (135, 34) -> (135, 33.7749) projected
  arc A50 (135, 33.7749) -> (136.7273, 33.0886) centre (136, 33.7749) ccw projected
  arc A51 (136.9114, 33.2727) -> (136.7273, 33.0886) centre (140, 30) ccw projected
  arc A52 (136.9114, 33.2727) -> (136.2251, 35) centre (136.2251, 34) ccw projected
  line L35 (136.2251, 35) -> (136, 35) projected
  arc A53 (136.7273, -167.2886) -> (135, -167.9749) centre (136, -167.9749) ccw projected
  line L36 (135, -167.9749) -> (135, -168.2) projected
  arc A54 (135, -168.2) -> (136, -169.2) centre (136, -168.2) ccw projected
  line L37 (136, -169.2) -> (136.2251, -169.2) projected
  arc A55 (136.2251, -169.2) -> (136.9114, -167.4727) centre (136.2251, -168.2) ccw projected
  arc A56 (136.7273, -167.2886) -> (136.9114, -167.4727) centre (140, -164.2) ccw projected
  line L38 (140.4377, -151.0763) -> (133.3836, -155.8731) projected
  arc A57 (133.3836, -155.8731) -> (133.3836, -157.5269) centre (133.9459, -156.7) ccw projected
  line L39 (133.3836, -157.5269) -> (137.0951, -160.0507) projected
  arc A58 (137.0951, -160.0507) -> (138.0834, -160.1286) centre (137.6574, -159.2238) ccw projected
  arc A59 (140.8182, -159.775) -> (138.0834, -160.1286) centre (140, -164.2) ccw projected
  arc A60 (140.8182, -159.775) -> (142, -158.7917) centre (141, -158.7917) ccw projected
  line L40 (142, -158.7917) -> (142, -151.9032) projected
  arc A61 (142, -151.9032) -> (140.4377, -151.0763) centre (141, -151.9032) ccw projected
  arc A62 (122.3542, 15.8269) -> (122.9165, 14) centre (122.9165, 15) ccw projected
  line L41 (122.9165, 14) -> (136.0835, 14) projected
  arc A63 (136.0835, 14) -> (136.6458, 15.8269) centre (136.0835, 15) ccw projected
  line L42 (136.6458, 15.8269) -> (130.0623, 20.3037) projected
  arc A64 (130.0623, 20.3037) -> (128.9377, 20.3037) centre (129.5, 19.4768) ccw projected
  line L43 (128.9377, 20.3037) -> (122.3542, 15.8269) projected
  arc A65 (125.6164, 21.6731) -> (125.6164, 23.3269) centre (125.0541, 22.5) ccw projected
  line L44 (125.6164, 23.3269) -> (118.5623, 28.1237) projected
  arc A66 (118.5623, 28.1237) -> (117, 27.2968) centre (118, 27.2968) ccw projected
  line L45 (117, 27.2968) -> (117, 17.7032) projected
  arc A67 (117, 17.7032) -> (118.5623, 16.8763) centre (118, 17.7032) ccw projected
  line L46 (118.5623, 16.8763) -> (125.6164, 21.6731) projected
  arc A68 (129.8, 31.1842) -> (133.4, 31.8) centre (131, 35) ccw projected
  arc A69 (129.8, 31.1842) -> (129.2, 31.1842) centre (129.5, 30.2303) ccw projected
  arc A70 (125.6, 31.8) -> (129.2, 31.1842) centre (128, 35) ccw projected
  arc A71 (125.6, 31.8) -> (125, 32) centre (125, 31) ccw projected
  line L47 (125, 32) -> (124, 32) projected
  line L48 (124, 32) -> (124, 34) projected
  arc A72 (124, 34) -> (123, 35) centre (123, 34) ccw projected
  line L49 (123, 35) -> (122, 35) projected
  arc A73 (122, 35) -> (121, 34) centre (122, 34) ccw projected
  line L50 (121, 34) -> (121, 32) projected
  arc A74 (121, 32) -> (120.7896, 30.237) centre (121.3519, 31.064) ccw projected
  line L51 (120.7896, 30.237) -> (128.9377, 24.6963) projected
  arc A75 (128.9377, 24.6963) -> (130.0623, 24.6963) centre (129.5, 25.5232) ccw projected
  line L52 (130.0623, 24.6963) -> (135.1564, 28.1603) projected
  arc A76 (135.1564, 28.1603) -> (135.577, 29.1713) centre (134.5941, 28.9872) ccw projected
  arc A77 (135.575, 30.8182) -> (135.577, 29.1713) centre (140, 30) ccw projected
  arc A78 (135.575, 30.8182) -> (134.5917, 32) centre (134.5917, 31) ccw projected
  line L53 (134.5917, 32) -> (134, 32) projected
  arc A79 (134, 32) -> (133.4, 31.8) centre (134, 31) ccw projected
  line L54 (118, 7) -> (118, 10) projected
  arc A80 (118, 10) -> (117, 11) centre (117, 10) ccw projected
  line L55 (117, 11) -> (96, 11) projected
  arc A81 (96, 11) -> (95, 10) centre (96, 10) ccw projected
  line L56 (95, 10) -> (95, 7) projected
  arc A82 (88.6, 3.8) -> (95, 7) centre (91, 7) ccw projected
  arc A83 (88.6, 3.8) -> (88, 4) centre (88, 3) ccw projected
  line L57 (88, 4) -> (87, 4) projected
  arc A84 (87, 4) -> (86.4, 3.8) centre (87, 3) ccw projected
  arc A85 (80.0808, 6.2) -> (86.4, 3.8) centre (84, 7) ccw projected
  arc A86 (80.0808, 6.2) -> (79.101, 7) centre (79.101, 6) ccw projected
  line L58 (79.101, 7) -> (64.5268, 7) projected
  arc A87 (64.5268, 7) -> (64.2705, 5.0334) centre (64.5268, 6) ccw projected
  line L59 (64.2705, 5.0334) -> (92.8926, -2.5553) projected
  arc A88 (92.8926, -2.5553) -> (93.4461, -2.5435) centre (93.1489, -1.5887) ccw projected
  line L60 (93.4461, -2.5435) -> (117.4252, 4.9211) projected
  arc A89 (117.4252, 4.9211) -> (118.1024, 6.1007) centre (117.128, 5.8759) ccw projected
  arc A90 (118, 7) -> (118.1024, 6.1007) centre (122, 7) ccw projected
  arc A91 (51, -14.398) -> (52.2972, -15.3528) centre (52, -14.398) ccw projected
  line L61 (52.2972, -15.3528) -> (84.4723, -5.337) projected
  arc A92 (84.4723, -5.337) -> (84.4313, -3.4155) centre (84.1751, -4.3821) ccw projected
  line L62 (84.4313, -3.4155) -> (52.2563, 5.1151) projected
  arc A93 (52.2563, 5.1151) -> (51, 4.1485) centre (52, 4.1485) ccw projected
  line L63 (51, 4.1485) -> (51, -14.398) projected
  arc A94 (63.1515, -117.2) -> (62.8561, -119.1554) centre (63.1515, -118.2) ccw projected
  line L64 (62.8561, -119.1554) -> (92.7876, -128.4114) projected
  arc A95 (92.7876, -128.4114) -> (93.3393, -128.4227) centre (93.0831, -127.4561) ccw projected
  line L65 (93.3393, -128.4227) -> (128.2505, -119.1666) projected
  arc A96 (128.2505, -119.1666) -> (127.9942, -117.2) centre (127.9942, -118.2) ccw projected
  line L66 (127.9942, -117.2) -> (63.1515, -117.2) projected
  arc A97 (132.8964, -140.2954) -> (133.575, -141.0246) centre (133.8705, -140.0692) ccw projected
  line L67 (133.575, -141.0246) -> (140.7046, -143.2293) projected
  arc A98 (140.7046, -143.2293) -> (142, -142.2739) centre (141, -142.2739) ccw projected
  line L68 (142, -142.2739) -> (142, -119.9245) projected
  arc A99 (142, -119.9245) -> (140.7437, -118.9579) centre (141, -119.9245) ccw projected
  line L69 (140.7437, -118.9579) -> (101.8327, -129.2745) projected
  arc A100 (101.8327, -129.2745) -> (101.7935, -131.1964) centre (102.089, -130.2411) ccw projected
  line L70 (101.7935, -131.1964) -> (121.1595, -137.1852) projected
  arc A101 (121.1595, -137.1852) -> (121.5639, -137.2238) centre (121.4549, -136.2298) ccw projected
  arc A102 (124.4, -138) -> (121.5639, -137.2238) centre (122, -141.2) ccw projected
  arc A103 (124.4, -138) -> (125, -138.2) centre (125, -137.2) ccw projected
  line L71 (125, -138.2) -> (126, -138.2) projected
  arc A104 (126, -138.2) -> (126.6, -138) centre (126, -137.2) ccw projected
  arc A105 (132.8964, -140.2954) -> (126.6, -138) centre (129, -141.2) ccw projected
  line L72 (83, -141.2) -> (83, -144.2) projected
  arc A106 (83, -144.2) -> (85, -144.2) centre (84, -144.2) ccw projected
  line L73 (85, -144.2) -> (90, -144.2) projected
  arc A107 (90, -144.2) -> (92, -144.2) centre (91, -144.2) ccw projected
  line L74 (92, -144.2) -> (92, -141.2) projected
  arc A108 (92, -141.2) -> (90, -141.2) centre (91, -141.2) ccw projected
  line L75 (90, -141.2) -> (85, -141.2) projected
  arc A109 (85, -141.2) -> (83, -141.2) centre (84, -141.2) ccw projected
  line L76 (121, 10) -> (121, 7) projected
  arc A110 (121, 7) -> (123, 7) centre (122, 7) ccw projected
  line L77 (123, 7) -> (128, 7) projected
  arc A111 (128, 7) -> (130, 7) centre (129, 7) ccw projected
  line L78 (130, 7) -> (130, 10) projected
  arc A112 (130, 10) -> (128, 10) centre (129, 10) ccw projected
  line L79 (128, 10) -> (123, 10) projected
  arc A113 (123, 10) -> (121, 10) centre (122, 10) ccw projected
  line L80 (85, 7) -> (90, 7) projected
  arc A114 (90, 7) -> (92, 7) centre (91, 7) ccw projected
  line L81 (92, 7) -> (92, 10) projected
  arc A115 (92, 10) -> (90, 10) centre (91, 10) ccw projected
  line L82 (90, 10) -> (85, 10) projected
  arc A116 (85, 10) -> (83, 10) centre (84, 10) ccw projected
  line L83 (83, 10) -> (83, 7) projected
  arc A117 (83, 7) -> (85, 7) centre (84, 7) ccw projected
  line L84 (123, -144.2) -> (128, -144.2) projected
  arc A118 (128, -144.2) -> (130, -144.2) centre (129, -144.2) ccw projected
  line L85 (130, -144.2) -> (130, -141.2) projected
  arc A119 (130, -141.2) -> (128, -141.2) centre (129, -141.2) ccw projected
  line L86 (128, -141.2) -> (123, -141.2) projected
  arc A120 (123, -141.2) -> (121, -141.2) centre (122, -141.2) ccw projected
  line L87 (121, -141.2) -> (121, -144.2) projected
  arc A121 (121, -144.2) -> (123, -144.2) centre (122, -144.2) ccw projected
  circle A122 centre (140, -164.2) radius 1.5 projected
  circle A123 centre (140, 30) radius 1.5 projected
  line L88 (48, 10) -> (79, 10) projected
  arc A124 (79, 10) -> (80, 11) centre (79, 11) ccw projected
  line L89 (80, 11) -> (80, 14) projected
  line L90 (80, 14) -> (113, 14) projected
  arc A125 (113, 14) -> (114, 15) centre (113, 15) ccw projected
  line L91 (114, 15) -> (114, 35) projected
  line L92 (114, 35) -> (116, 35) projected
  arc A126 (116, 35) -> (118, 35) centre (117, 35) ccw projected
  line L93 (118, 35) -> (118, 38) projected
  line L94 (118, 38) -> (127, 38) projected
  line L95 (127, 38) -> (127, 35) projected
  arc A127 (127, 35) -> (129, 35) centre (128, 35) ccw projected
  line L96 (129, 35) -> (130, 35) projected
  arc A128 (130, 35) -> (132, 35) centre (131, 35) ccw projected
  line L97 (132, 35) -> (132, 38) projected
  line L98 (132, 38) -> (141, 38) projected
  line L99 (141, 38) -> (141, 35) projected
  arc A129 (141, 35) -> (143, 35) centre (142, 35) ccw projected
  line L100 (143, 35) -> (145, 35) projected
  line L101 (145, 35) -> (145, -169.2) projected
  line L102 (145, -169.2) -> (143, -169.2) projected
  arc A130 (143, -169.2) -> (141, -169.2) centre (142, -169.2) ccw projected
  line L103 (141, -169.2) -> (141, -172.2) projected
  line L104 (141, -172.2) -> (132, -172.2) projected
  line L105 (132, -172.2) -> (132, -169.2) projected
  arc A131 (132, -169.2) -> (130, -169.2) centre (131, -169.2) ccw projected
  line L106 (130, -169.2) -> (129, -169.2) projected
  arc A132 (129, -169.2) -> (127, -169.2) centre (128, -169.2) ccw projected
  line L107 (127, -169.2) -> (127, -172.2) projected
  line L108 (127, -172.2) -> (118, -172.2) projected
  line L109 (118, -172.2) -> (118, -169.2) projected
  arc A133 (118, -169.2) -> (116, -169.2) centre (117, -169.2) ccw projected
  line L110 (116, -169.2) -> (114, -169.2) projected
  line L111 (114, -169.2) -> (114, -149.2) projected
  arc A134 (114, -149.2) -> (113, -148.2) centre (113, -149.2) ccw projected
  line L112 (113, -148.2) -> (80, -148.2) projected
  line L113 (80, -148.2) -> (80, -145.2) projected
  arc A135 (80, -145.2) -> (79, -144.2) centre (79, -145.2) ccw projected
  line L114 (79, -144.2) -> (48, -144.2) projected
  line L115 (48, -144.2) -> (48, 10) projected
  line L116 (51, -111.2) -> (142, -111.2)
  line L117 (145, -169.2) -> (145, 35) projected
  line L118 (51, -23) -> (142, -23)
  line L119 (145, 32) -> (144.6458, 32)
  arc A136 (138, 35) -> (144.6458, 32) centre (142, 35) ccw
  line L120 (138, 35) -> (135, 35)
  arc A137 (129.5, 38.7081) -> (135, 35) centre (131, 35) ccw
  arc A138 (124, 35) -> (129.5, 38.7081) centre (128, 35) ccw
  line L121 (124, 35) -> (121, 35)
  arc A139 (117, 39) -> (121, 35) centre (117, 35) ccw
  line L122 (117, 39) -> (117, 15)
  arc A140 (113, 11) -> (117, 15) centre (113, 15) ccw
  line L123 (113, 11) -> (83, 11)
  arc A141 (79, 7) -> (83, 11) centre (79, 11) ccw
  line L124 (79, 7) -> (51, 7)
  line L125 (51, -141.2) -> (79, -141.2)
  arc A142 (83, -145.2) -> (79, -141.2) centre (79, -145.2) ccw
  line L126 (83, -145.2) -> (113, -145.2)
  arc A143 (117, -149.2) -> (113, -145.2) centre (113, -149.2) ccw
  line L127 (117, -149.2) -> (117, -173.2)
  arc A144 (121, -169.2) -> (117, -173.2) centre (117, -169.2) ccw
  line L128 (121, -169.2) -> (124, -169.2)
  arc A145 (129.5, -165.4919) -> (124, -169.2) centre (128, -169.2) ccw
  arc A146 (135, -169.2) -> (129.5, -165.4919) centre (131, -169.2) ccw
  line L129 (135, -169.2) -> (138, -169.2)
  arc A147 (144.6458, -166.2) -> (138, -169.2) centre (142, -169.2) ccw
  line L130 (144.6458, -166.2) -> (145, -166.2)
  line L131 (51, -119.9851) -> (51, -141.2)
  line L132 (142, -119.9245) -> (142, -169.2)
  line L133 (142, 35) -> (142, -14.2755)
  line L134 (142, -23) -> (142, -111.2)
  line L135 (51, 7) -> (51, -14.398)
  line L136 (51, -23) -> (51, -111.2)
  point P0 (0, 0)
  dimension "d8" = 6
  dimension "d9" = 6
  constraints: 40 end point, 28 point on circle, 12 centre point, 3 parallel, 2 perpendicular, 22 other
  measures "d8" distance between parallel lines of L118 L6
  measures "d9" distance between parallel lines of L116 L66
extrude "押し出し3" cut sketch "スケッチ4" against normal blind 1.5 contours L136 L118 L134 L116
bend part "曲げパーツ1" radius 1 angle 90 line through (48, -114.2, 2) along (1, 0, 0) centre toward (0, 0, 1) moving side (0, -1, 0) both sides no
bend part "曲げパーツ2" radius 1 angle 90 line through (48, -20, 2) along (1, 0, 0) centre toward (0, 0, 1) moving side (0, 1, 0) both sides no
equation "\"d7\" = d6"
